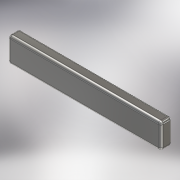
# Autodesk Inventor part: Magnet6010
Saved by Autodesk Inventor 2018 (Build 220112000, 112)
## iProperties
Created: 2018-03-25
Part Number: Magnet6010
Material: Stainless Steel
Document SubType Name: Modeling
Designer: mansu
Density: 8 g/cm^3
Appearance: Chrome - Polished
Author: mansu
Autodesk Inventor part; units mm, degrees
ref_plane "YZ Plane" through (0, 0, 0) normal (1, 0, 0) x (0, 1, 0)
ref_plane "XZ Plane" through (0, 0, 0) normal (0, 1, 0) x (-1, 0, 0)
ref_plane "XY Plane" through (0, 0, 0) normal (0, 0, 1) x (1, 0, 0)
sketch "Sketch1" plane through (0, 0, 0) normal (0, 1, 0) x (-1, 0, 0)
  line L0 (0, 0) -> (-58, 0)
  line L1 (-58, 0) -> (-58, -9.5)
  line L2 (-58, -9.5) -> (0, -9.5)
  line L3 (0, -9.5) -> (0, 0)
  dimension "d0" = 58
  dimension "d1" = 9.5
  constraints: 8 end point, 2 parallel, 1 horizontal, 1 perpendicular
  measures "d0" distance of L2.end L1.end
  measures "d1" distance of L1.end L0.end
extrude "Extrusion1" add sketch "Sketch1" along normal blind 4.3
fillet "Fillet1" radius 1 12 edges at (0, 0, -4.75) (0, 2.15, 0) (0, 4.3, -4.75) (0, 2.15, -9.5) (29, 0, -9.5) (29, 4.3, -9.5) (58, 2.15, -9.5) (58, 0, -4.75) (58, 4.3, -4.75) (58, 2.15, 0) (29, 0, 0) (29, 4.3, 0)
body "Solid1"
